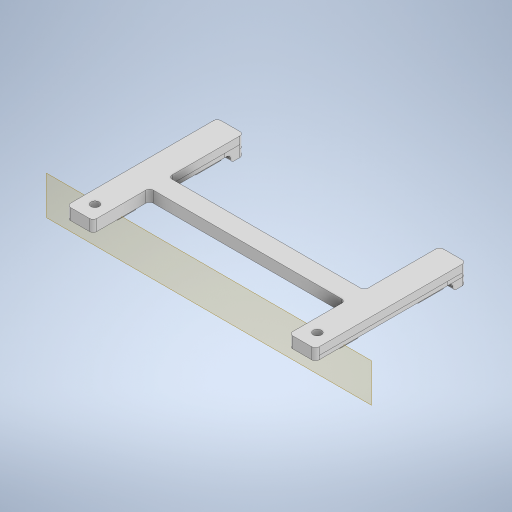
# Autodesk Inventor part: _Wallmount
Saved by Autodesk Inventor 2024.3 (Build 283343000, 343)
## iProperties
Created: 2024-10-18
Part Number: _Wallmount
Material: Generic
Document SubType Name: Modeling
Designer: atrus
Density: 1 g/cm^3
Appearance: Default
Author: atrus
Autodesk Inventor part; units mm, degrees
ref_plane "YZ Plane" through (0, 0, 0) normal (1, 0, 0) x (0, 1, 0)
ref_plane "XZ Plane" through (0, 0, 0) normal (0, 1, 0) x (-1, 0, 0)
ref_plane "Work Plane1" through (0, 0, 0) normal (0, 0, 1) x (1, 0, 0)
sketch "Sketch1" plane through (0, 0, 0) normal (0, 0, 1) x (1, 0, 0)
  line L0 (-137.5, 4) -> (-135.5, 6) construction
  line L1 (-126.5, 4) -> (-137.5, 4) construction
  line L2 (-128.5, 6) -> (-126.5, 4) construction
  line L3 (-10.5, 6) -> (-8.5, 4) construction
  line L4 (-8.5, 4) -> (-19.5, 4) construction
  line L5 (-19.5, 4) -> (-17.5, 6) construction
  line L6 (-17.3586, 5.8586) -> (-19.0171, 4.2)
  line L7 (-19.0171, 4.2) -> (-8.9828, 4.2)
  line L8 (-8.9828, 4.2) -> (-10.6414, 5.8586)
  line L9 (-128.7828, 6) -> (-126.9828, 4.2)
  line L10 (-126.9828, 4.2) -> (-137.0171, 4.2)
  line L11 (-137.0171, 4.2) -> (-135.2171, 6)
  line L12 (-128.7828, 6) -> (-128.7828, 6.5)
  line L13 (-128.7828, 6.5) -> (-125, 6.5)
  line L14 (-125, 6.5) -> (-125, 8.5)
  line L15 (-125, 8.5) -> (-139, 8.5)
  line L16 (-139, 8.5) -> (-139, 6.5)
  line L17 (-139, 6.5) -> (-135.2171, 6.5)
  line L18 (-135.2171, 6.5) -> (-135.2171, 6)
  line L19 (-17.5, 6) -> (-128.5, 6) construction
  line L20 (-73, 6) -> (-73, 54.8085) construction
  line L21 (-17.2171, 6) -> (-17.2171, 6.5)
  line L22 (-17.2171, 6.5) -> (-21, 6.5)
  line L23 (-21, 6.5) -> (-21, 8.5)
  line L24 (-21, 8.5) -> (-7, 8.5)
  line L25 (-7, 8.5) -> (-7, 6.5)
  line L26 (-7, 6.5) -> (-10.7828, 6.5)
  line L27 (-10.7828, 6.5) -> (-10.7828, 6)
  line L28 (-17.3586, 5.8586) -> (-17.2171, 6)
  line L29 (-10.6414, 5.8586) -> (-10.7828, 6)
  point P0 (0, 0)
  point P1 (-132, 4)
  point P2 (-132, 4.2)
  point P3 (-14, 4)
  point P4 (-14, 4.2)
  dimension "d0" = 0.2
  dimension "d1" = 0.2
  dimension "d2" = 2
  dimension "d3" = 14
  dimension "d4" = 0.5
  dimension "d5" = 0.5
  constraints: 48 end point, 8 symmetric about line, 6 perpendicular, 5 midpoint, 4 point on line, 2 equal length, 2 vertical, 1 horizontal, 4 other
  measures "d0" distance of point (-132, 4) point (-132, 4.2)
  measures "d1" distance of point (-14, 4) point (-14, 4.2)
  measures "d2" distance of L15.end L16.end
  measures "d3" distance of L14.end L15.end
  measures "d4" distance of L9.start L12.end
  measures "d5" distance from line of L0.end L17
ref_plane "Work Plane2" through (-157, -12.598, -54.9) normal (-0.0000001, 0, -1) x (0, 1, 0)
extrude "Extrusion1" add sketch "Sketch1" against normal up to surface (54.9 mm away)
sketch "Sketch2" plane through (-7, 8.5, -54.9) normal (-0.0000001, 0, -1) x (-1, 0, 0.0000001)
  line L0 (0, 0) -> (14, 0) projected
  line L1 (3.7828, -2) -> (0, -2) projected
  line L2 (14, 0) -> (0, 0)
  line L3 (0, 0) -> (0, -2)
  line L4 (0, -2) -> (14, -2)
  line L5 (14, -2) -> (14, 0)
  line L6 (118, -2) -> (118, 0) projected
  line L7 (132, 0) -> (118, 0)
  line L8 (118, 0) -> (118, -2)
  line L9 (118, -2) -> (132, -2)
  line L10 (132, -2) -> (132, 0)
  point P0 (-7, -8.5)
  point P1 (118, 0)
  point P2 (0, 0)
  constraints: 16 end point, 4 parallel, 2 horizontal, 2 perpendicular, 1 coincident, 1 point on line
extrude "Extrusion2" add sketch "Sketch2" along normal blind 10
sketch "Sketch3" plane through (-139, 6.5, 0) normal (0, -1, 0) x (1, 0, 0)
  line L0 (14, -54.9) -> (14, -64.9) projected
  line L1 (0, -54.9) -> (0, -64.9) projected
  line L2 (14, -64.9) -> (0, -64.9)
  line L3 (0, -64.9) -> (0, -57.9)
  line L4 (0, -57.9) -> (14, -57.9)
  line L5 (14, -57.9) -> (14, -64.9)
  line L6 (132, -64.9) -> (118, -64.9) projected
  line L7 (132, -54.9) -> (132, -64.9) projected
  line L8 (118, -64.9) -> (132, -64.9)
  line L9 (132, -64.9) -> (132, -57.9)
  line L10 (132, -57.9) -> (118, -57.9)
  line L11 (118, -57.9) -> (118, -64.9)
  point P0 (139, 0)
  point P1 (14, -57.9)
  dimension "d10" = 7
  dimension "d11" = 7
  constraints: 16 end point, 4 parallel, 2 horizontal, 2 perpendicular, 2 point on line
  measures "d10" distance between parallel lines of L2 L4
  measures "d11" distance of L8.end L9.end
extrude "Extrusion3" add sketch "Sketch3" along normal blind 4
fillet "Fillet1" radius 2 4 edges at (-132, 2.5, -57.9) (-14, 2.5, -57.9) (-132, 6.5, -57.9) (-14, 6.5, -57.9)
sketch "Sketch4" plane through (0, 0, 0) normal (0, 0, 1) x (1, 0, 0)
  line L0 (-7, 8.5) -> (-7, 6.5) projected
  line L1 (-21, 6.5) -> (-21, 8.5) projected
  line L2 (-7, 8.5) -> (-21, 8.5)
  line L3 (-21, 8.5) -> (-21, 6.5)
  line L4 (-21, 6.5) -> (-7, 6.5)
  line L5 (-7, 6.5) -> (-7, 8.5)
  line L6 (-139, 6.5) -> (-139, 8.5) projected
  line L7 (-125, 6.5) -> (-125, 8.5) projected
  line L8 (-139, 6.5) -> (-125, 6.5)
  line L9 (-125, 6.5) -> (-125, 8.5)
  line L10 (-125, 8.5) -> (-139, 8.5)
  line L11 (-139, 8.5) -> (-139, 6.5)
  point P0 (0, 0)
  constraints: 16 end point, 4 parallel, 2 horizontal, 2 perpendicular
extrude "Extrusion4" add sketch "Sketch4" along normal blind 15
sketch "Sketch5" plane through (-139, 6.5, -55.9) normal (0, -1, 0) x (1, 0, 0)
  line L0 (0, 70.9) -> (14, 70.9) construction
  line L1 (7, 70.9) -> (7, 62.9) construction
  line L2 (118, 70.9) -> (132, 70.9) construction
  line L3 (125, 70.9) -> (125, 62.9) construction
  point P0 (139, 55.9)
  dimension "d17" = 8
  constraints: 4 end point, 2 coincident, 2 midpoint, 2 vertical, 1 parallel
  measures "d17" distance of L1.start L1.end
hole "Hole1" at (-132, 6.5, 7) at (-14, 6.5, 7) direction (0, 1, 0) diameter 4.318 end through all countersink diameter 7.0866 countersink angle 82 clearance for "Flat Head Machine Screw (82)" size "#6" standard "Ansi Unified Screw Threads"
sketch "Sketch6" plane through (-139, 8.5, -64.9) normal (0, 1, 0) x (1, 0, -0.0000001)
  line L0 (118, -39.95) -> (14, -39.95)
  line L1 (14, -39.95) -> (14, -49.95)
  line L2 (14, -49.95) -> (118, -49.95)
  line L3 (118, -49.95) -> (118, -39.95)
  line L4 (118, -10) -> (118, -79.9) projected
  line L5 (14, -10) -> (14, -79.9) projected
  point P0 (139, -64.9)
  point P1 (118, -44.95)
  point P2 (14, -44.95)
  dimension "d26" = 10
  constraints: 8 end point, 4 midpoint, 2 parallel, 1 horizontal, 1 perpendicular
  measures "d26" distance of L2.end L0.start
extrude "Extrusion5" add sketch "Sketch6" against normal up to surface (2 mm away)
fillet "Fillet2" radius 2 16 edges at (-21, 7.5, -14.95) (-21, 7.5, -24.95) (-125, 7.5, -24.95) (-125, 7.5, -14.95) (-125, 7.5, 15) (-139, 7.5, 15) (-21, 7.5, 15) (-7, 7.5, 15) (-7, 5.5, -64.9) (-21, 7.5, -64.9) (-21, 4.5, -64.9) (-14, 2.5, -64.9) (-125, 4.5, -64.9) (-125, 7.5, -64.9) (-132, 2.5, -64.9) (-139, 5.5, -64.9)
sketch "Sketch7" plane through (-139, 6.5, -54.9) normal (-1, 0, 0) x (0, 0, 1)
  line L0 (14.44, -0.5) -> (14.44, -2.5) construction
  line L1 (44.25, -2.5) -> (44.25, -0.5) construction
  line L2 (54.9, -2.3) -> (0, -2.3) projected
  line L3 (13.44, 0) -> (45.25, 0)
  line L4 (45.25, 0) -> (45.25, -2.3)
  line L5 (45.25, -2.3) -> (13.44, -2.3)
  line L6 (13.44, -2.3) -> (13.44, 0)
  line L7 (0, 0) -> (67.9, 0) construction
  line L8 (27.95, 0) -> (0, 0) projected
  point P0 (54.9, -6.5)
  point P1 (13.975, 0)
  point P2 (44.25, -1.5)
  point P3 (13.44, -2.3)
  dimension "d30" = 1
  dimension "d31" = 1
  constraints: 10 end point, 2 midpoint, 2 parallel, 2 point on line, 1 horizontal, 1 perpendicular, 1 vertical, 2 other
  measures "d30" distance between parallel lines of L6 L0
  measures "d31" distance from line of point (44.25, -1.5) L4
extrude "Extrusion6" cut sketch "Sketch7" against normal through all
chamfer "Chamfer1" distance 2 angle 45 4 edges at (-132, 6.5, -41.46) (-14, 6.5, -41.46) (-132, 6.5, 0) (-14, 6.5, 0)
sketch "Sketch8" plane through (-7, 8.5, 0) normal (0, 1, 0) x (1, 0, 0)
  arc A0 (-130, 64.9) -> (-132, 62.9) centre (-130, 62.9) ccw projected
  line L0 (-132, 54.9) -> (-132, 62.9) projected
  line L1 (-132, 54.9) -> (-132, -13) projected
  arc A1 (-132, -13) -> (-130, -15) centre (-130, -13) ccw projected
  line L2 (-120, -15) -> (-130, -15) projected
  arc A2 (-120, -15) -> (-118, -13) centre (-120, -13) ccw projected
  line L3 (-118, 12.95) -> (-118, -13) projected
  arc A3 (-116, 14.95) -> (-118, 12.95) centre (-116, 12.95) ccw projected
  line L4 (-116, 14.95) -> (-16, 14.95) projected
  arc A4 (-14, 12.95) -> (-16, 14.95) centre (-16, 12.95) ccw projected
  line L5 (-14, 12.95) -> (-14, -13) projected
  arc A5 (-14, -13) -> (-12, -15) centre (-12, -13) ccw projected
  line L6 (-2, -15) -> (-12, -15) projected
  arc A6 (-2, -15) -> (0, -13) centre (-2, -13) ccw projected
  line L7 (0, 0) -> (0, -13) projected
  line L8 (0, 0) -> (0, 54.9) projected
  line L9 (0, 54.9) -> (0, 62.9) projected
  arc A7 (0, 62.9) -> (-2, 64.9) centre (-2, 62.9) ccw projected
  line L10 (-12, 64.9) -> (-2, 64.9) projected
  arc A8 (-12, 64.9) -> (-14, 62.9) centre (-12, 62.9) ccw projected
  line L11 (-14, 54.9) -> (-14, 62.9) projected
  line L12 (-14, 54.9) -> (-14, 26.95) projected
  arc A9 (-16, 24.95) -> (-14, 26.95) centre (-16, 26.95) ccw projected
  line L13 (-16, 24.95) -> (-116, 24.95) projected
  arc A10 (-118, 26.95) -> (-116, 24.95) centre (-116, 26.95) ccw projected
  line L14 (-118, 54.9) -> (-118, 26.95) projected
  line L15 (-118, 54.9) -> (-118, 62.9) projected
  arc A11 (-118, 62.9) -> (-120, 64.9) centre (-120, 62.9) ccw projected
  line L16 (-130, 64.9) -> (-120, 64.9) projected
  circle A12 centre (-125, -7) radius 2.159 projected
  circle A13 centre (-7, -7) radius 2.159 projected
  point P0 (7, 0)
extrude "Extrusion7" add sketch "Sketch8" along normal blind 4
body "Solid1"
